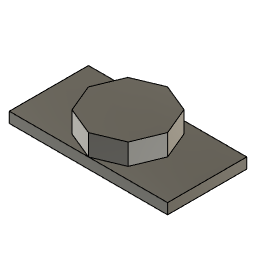
stopSignPiece (Autodesk Fusion 360 archive; units mm, degrees)
design "stopSign" references "TactileMapsParameters"
Autodesk Fusion 360 part; units mm, degrees
derive "ExternalDerived1" from "TactileMapsParameters v7"
sketch "Sketch1" plane through (0, 0, 0) normal (0, 0, 1) x (1, 0, 0)
  line L0 (0, 0) -> (12, 0)
  line L1 (12, 0) -> (12, 6)
  line L2 (12, 6) -> (0, 6)
  line L3 (0, 6) -> (0, 0)
  dimension "d18" = 12
  dimension "d19" = 6
  constraint horizontal L0
  constraint vertical L1
  constraint horizontal L2
  constraint vertical L3
  constraint coincident L0.start L3.end
  measures "d18" distance of L0.start L0.end
  measures "d19" distance of L0.start L2.end
extrude "Extrude1" add sketch "Sketch1" along normal blind 0.8
sketch "Sketch2" plane through (0, 0, 0.8) normal (0, 0, 1) x (-1, 0, 0)
  line L0 (0, -6) -> (0, 0)
  line L1 (0, 0) -> (-12, 0)
  line L2 (-12, 0) -> (-12, -6)
  line L3 (-12, -6) -> (0, -6)
  line L4 (0, -3) -> (-12.0141, -3) construction
  line L5 (-6, -6) -> (-6, 0) construction
  line L6 (-8.1153, -5.1273) -> (-5.9915, -6)
  line L7 (-5.9915, -6) -> (-3.8727, -5.1153)
  line L8 (-3.8727, -5.1153) -> (-3, -2.9915)
  line L9 (-3, -2.9915) -> (-3.8847, -0.8727)
  line L10 (-3.8847, -0.8727) -> (-6.0085, 0)
  line L11 (-6.0085, 0) -> (-8.1273, -0.8847)
  line L12 (-8.1273, -0.8847) -> (-9, -3.0085)
  line L13 (-9, -3.0085) -> (-8.1153, -5.1273)
  line L14 (0, -6) -> (0, 0)
  line L15 (0, 0) -> (-12, 0)
  line L16 (-12, 0) -> (-12, -6)
  line L17 (-12, -6) -> (0, -6)
  point P0 (-6, -3)
  point P1 (-6, -3)
  dimension "d24" = 3
  constraint midpoint L0 L4.start
  constraint perpendicular L2 L4
  constraint midpoint L3 L5.start
  constraint midpoint L1 L5.end
  constraint midpoint L5 P1
  constraint coincident P1 P0
  measures "d24" distance of L6.start P1
extrude "Extrude3" add sketch "Sketch2" along normal blind 1.6 contours L6 L7 L8 L9 L10 L11 L12 L13
equation "length_Ref = 170 mm" comment "Side lengths of base of model"
equation "baseHeight_Ref = 0.4 mm" comment "Height of the base of the model"
equation "sidewalkHeight_Ref = 3.2 mm" comment "Height of sidewalk/walking surface"
equation "sidewalkWidth_Ref = length_Ref / 3" comment "Width of the sidewalk/walking surface"
equation "orientorSize_Ref = 6 mm" comment "Side length of orientation indicator square"
equation "oritentorHeight_Ref = 2.4 mm" comment "Height of the orientation indicator"
equation "braileHeight_Ref = 0.6 mm" comment "Standard height of Braille characters"
equation "filletRadius_Ref = 0.6 mm" comment "Radius of fillets to soften edges"
equation "lineWidth_Ref = 3 mm" comment "Width of crosswalk lines"
equation "lineHeight_Ref = braileHeight_Ref / 2" comment "Height of crosswalk lines"
equation "tabWidth_Ref = length_Ref / 10" comment "Width of tabs to secure adjacent maps together"
equation "tabLength_Ref = length_Ref / 14" comment "Length of tab to secure adjacent maps together"
equation "tabHeight_Ref = sidewalkHeight_Ref / 4" comment "Height of tabs to secure adjacent maps together"
equation "clearance_Ref = 0.2 mm" comment "Clearance around parts that will fit together"
equation "featureHeight_Ref = 1.6 mm" comment "Height of features such as bus stops"
equation "pegSize_Ref = 6 mm" comment "Side length of pegs/holes to connect features to map base"
equation "pegDepth_Ref = sidewalkHeight_Ref / 4" comment "Depth of pegs/holes to connect features to map base"
equation "d18 = 2 * pegSize_Ref"
equation "d19 = pegSize_Ref"
equation "d20 = pegDepth_Ref"
equation "d24 = pegSize_Ref / 2"
equation "d25 = featureHeight_Ref"
equation "dogbone_Ref = 2 mm" comment "\"Cutter\" diameter for creating dogbone corners."
